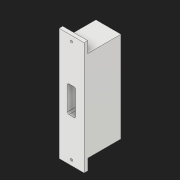
# Autodesk Inventor part: BP005
Saved by Autodesk Inventor 2017 SP1 (Build 210196100, 196)
## iProperties
Created: 2018-01-07
Part Number: BP005
Material: ABS Plastic
Document SubType Name: Modeling
Designer: Zach
Density: 1.06 g/cm^3
Appearance: CR White
Author: Zach
Autodesk Inventor part; units mm, degrees
ref_plane "YZ Plane" through (0, 0, 0) normal (1, 0, 0) x (0, 1, 0)
ref_plane "XZ Plane" through (0, 0, 0) normal (0, 1, 0) x (-1, 0, 0)
ref_plane "XY Plane" through (0, 0, 0) normal (0, 0, 1) x (1, 0, 0)
sketch "Sketch1" plane through (0, 0, 0) normal (0, 0, 1) x (1, 0, 0)
  line L0 (0, 0) -> (34, 0)
  line L1 (34, 0) -> (34, 153)
  line L2 (34, 153) -> (0, 153)
  line L3 (0, 153) -> (0, 0)
  circle A0 centre (17, 7) radius 1.5
  circle A1 centre (17, 146) radius 1.5
  point P0 (17, 153)
  point P1 (17, 0)
  dimension "d0" = 34
  dimension "d1" = 153
  dimension "d2" = 3
  dimension "d4" = 7
  dimension "d5" = 3
  dimension "d6" = 7
  constraints: 8 end point, 2 centre point, 2 midpoint, 2 parallel, 2 vertical alignment, 1 horizontal, 1 perpendicular
  measures "d0" distance of L2.end L1.end
  measures "d1" distance of L1.end L0.end
  measures "d2" diameter of A0
  measures "d4" distance from line of L0 A0.centre
  measures "d5" diameter of A1
  measures "d6" distance from line of L2 A1.centre
extrude "Extrusion1" add sketch "Sketch1" along normal blind 5
sketch "Sketch2" plane through (0, 0, 0) normal (0, 0, -1) x (-1, 0, 0)
  line L0 (0, 153) -> (0, 0) projected
  line L1 (0, 138) -> (-34, 138)
  line L2 (-34, 138) -> (-34, 15)
  line L3 (-34, 15) -> (0, 15)
  line L4 (0, 15) -> (0, 138)
  line L5 (-34, 0) -> (-34, 153) projected
  point P0 (0, 76.5)
  dimension "d10" = 123
  constraints: 8 end point, 2 midpoint, 2 parallel, 2 point on line, 1 horizontal, 1 perpendicular
  measures "d10" distance of L2.end L1.end
extrude "Extrusion2" add sketch "Sketch2" along normal blind 5
sketch "Sketch7" plane through (0, 0, 5) normal (0, 0, 1) x (1, 0, 0)
  line L0 (22.5, 94.5) -> (11.5, 94.5)
  line L1 (11.5, 94.5) -> (11.5, 58.5)
  line L2 (11.5, 58.5) -> (22.5, 58.5)
  line L3 (22.5, 58.5) -> (22.5, 94.5)
  line L4 (34, 0) -> (34, 153) projected
  line L5 (34, 153) -> (0, 153) projected
  point P0 (0, 0)
  point P1 (22.5, 76.5)
  point P2 (34, 76.5)
  point P3 (17, 58.5)
  point P4 (17, 153)
  dimension "d26" = 36
  dimension "d27" = 11
  constraints: 8 end point, 4 midpoint, 2 parallel, 1 horizontal, 1 horizontal alignment, 1 perpendicular, 1 vertical alignment
  measures "d26" distance of L2.end L0.start
  measures "d27" distance of L1.end L2.end
extrude "Extrusion5" cut sketch "Sketch7" against normal through all
fillet "Fillet1" radius 2 4 edges at (22.5, 94.5, 0) (11.5, 94.5, 0) (22.5, 58.5, 0) (11.5, 58.5, 0)
sketch "Sketch8" plane through (0, 0, -5) normal (0, 0, -1) x (-1, 0, 0)
  line L0 (-11.5, 92.5) -> (-11.5, 60.5) projected
  arc A0 (-13.5, 58.5) -> (-11.5, 60.5) centre (-13.5, 60.5) ccw projected
  line L1 (-13.5, 58.5) -> (-20.5, 58.5) projected
  arc A1 (-22.5, 60.5) -> (-20.5, 58.5) centre (-20.5, 60.5) ccw projected
  line L2 (-22.5, 60.5) -> (-22.5, 92.5) projected
  arc A2 (-20.5, 94.5) -> (-22.5, 92.5) centre (-20.5, 92.5) ccw projected
  line L3 (-20.5, 94.5) -> (-13.5, 94.5) projected
  arc A3 (-11.5, 92.5) -> (-13.5, 94.5) centre (-13.5, 92.5) ccw projected
  line L4 (0, 138) -> (-34, 138) projected
  line L5 (-34, 138) -> (-34, 15) projected
  line L6 (-34, 15) -> (0, 15) projected
  line L7 (0, 15) -> (0, 138) projected
  point P0 (0, 0)
extrude "Extrusion6" add sketch "Sketch8" along normal blind 40
body "Solid1"
